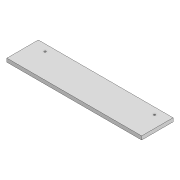
# Autodesk Inventor part: Wing_base
Saved by Autodesk Inventor 2022 (Build 260153000, 153)
## iProperties
Created: 2022-07-07
Part Number: Wing_base
Material: Generic
Document SubType Name: Modeling
Designer: dell
Density: 1 g/cm^3
Appearance: Default
Author: dell
Autodesk Inventor part; units mm, degrees
ref_plane "YZ Plane" through (0, 0, 0) normal (1, 0, 0) x (0, 1, 0)
ref_plane "XZ Plane" through (0, 0, 0) normal (0, 1, 0) x (-1, 0, 0)
ref_plane "XY Plane" through (0, 0, 0) normal (0, 0, 1) x (1, 0, 0)
sketch "Sketch1" plane through (0, 0, 0) normal (0, 1, 0) x (-1, 0, 0)
  line L0 (0, 0) -> (300, 0)
  line L1 (300, 0) -> (300, -70)
  line L2 (300, -70) -> (0, -70)
  line L3 (0, -70) -> (0, 0)
  circle A0 centre (270, -55) radius 2
  circle A1 centre (26.349, -55) radius 2
  dimension "d0" = 300
  dimension "d1" = 70
  dimension "d2" = 4
  dimension "d3" = 4
  dimension "d4" = 243.651
  dimension "d5" = 30
  dimension "d6" = 15
  dimension "d7" = 15
  constraints: 8 end point, 2 centre point, 2 parallel, 1 horizontal, 1 perpendicular
  measures "d0" distance of L1.end L2.end
  measures "d1" distance of L2.end L0.start
  measures "d2" diameter of A0
  measures "d3" diameter of A1
  measures "d4" distance of A1.centre A0.centre
  measures "d5" distance from line of L1 A0.centre
  measures "d6" distance from line of L2 A0.centre
  measures "d7" distance from line of L2 A1.centre
extrude "Extrusion1" add sketch "Sketch1" along normal blind 8
equation "\"d7\" = d6"
body "Solid1"
